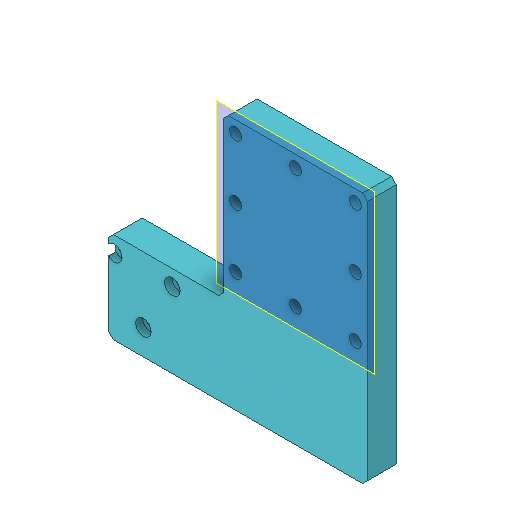
# Autodesk Inventor part: cellSTORM_Base_v0_R1
Saved by Autodesk Inventor 2022 (Build 260153000, 153)
## iProperties
Created: 2019-10-29
Part Number: cellSTORM_Base_v0_R1
Material: Generic
Document SubType Name: Modeling
Designer: diederichbenedict
Density: 1 g/cm^3
Appearance: Default
Sheet Metal Rule: Standard
Author: diederichbenedict
Autodesk Inventor part; units mm, degrees
ref_plane "YZ Plane" through (0, 0, 0) normal (1, 0, 0) x (0, 1, 0)
ref_plane "XZ Plane" through (0, 0, 0) normal (0, 1, 0) x (-1, 0, 0)
ref_plane "XY Plane" through (0, 0, 0) normal (0, 0, 1) x (1, 0, 0)
ref_plane "Arbeitsebene2" through (0, 0, 0) normal (0, 0, -1) x (0, 1, 0)
sketch "Skizze6" plane through (0, 0, 0) normal (0, 0, -1) x (0, 1, 0)
  circle A0 centre (0, 25) radius 1.95 projected
  circle A1 centre (-25, 0) radius 1.95 projected
  circle A2 centre (-25, -25) radius 1.95 projected
  circle A3 centre (25, 25) radius 1.95 projected
  circle A4 centre (25, -25) radius 1.95 projected
  circle A5 centre (-25, 25) radius 1.95 projected
  circle A6 centre (25, 0) radius 1.95 projected
  circle A7 centre (0, -25) radius 1.95 projected
  line L0 (-28, 30) -> (-30, 28) projected
  line L1 (-30, 28) -> (-30, -28) projected
  line L2 (-30, -28) -> (-28, -30) projected
  line L3 (-28, -30) -> (28, -30) projected
  line L4 (28, -30) -> (30, -28) projected
  line L5 (30, -28) -> (30, 28) projected
  line L6 (30, 28) -> (28, 30) projected
  line L7 (28, 30) -> (-28, 30) projected
  line L8 (-40.5166, -48.4344) -> (-70.5166, -48.4344) construction
  line L9 (-70.5166, -48.4344) -> (-70.5166, -78.4344) construction
  line L10 (-70.5166, -78.4344) -> (-40.5166, -78.4344) construction
  line L11 (-40.5166, -78.4344) -> (-40.5166, -48.4344) construction
  line L12 (-40.5166, -48.4344) -> (-70.5166, -78.4344) construction
  line L13 (-70.5166, -48.4344) -> (-40.5166, -78.4344) construction
  line L14 (-75, -48) -> (-45, -48)
  line L15 (-45, -48) -> (-45, -78)
  line L16 (-45, -78) -> (-75, -78)
  line L17 (-75, -78) -> (-75, -48)
  line L18 (-75, -48) -> (-45, -78) construction
  line L19 (-45, -48) -> (-75, -78) construction
  line L20 (-45, -48) -> (-30, -48)
  line L21 (-30, -48) -> (-30, -28)
  line L22 (-45, -78) -> (0, -78)
  line L23 (0, -78) -> (0, -30)
  circle A8 centre (-55.5095, -63.317) radius 8.4793 projected
  line L24 (-28, 30) -> (-75, 30)
  line L25 (-75, 30) -> (-75, -48)
  line L26 (-28, -30) -> (-45, -30)
  line L27 (-45, -30) -> (-45, -48)
  line L28 (-45, -78) -> (-37, -78)
  line L29 (-37, -78) -> (-37, -48)
  line L30 (-37, -48) -> (-45, -48)
  line L31 (-45, -48) -> (-45, -78)
  line L32 (-45, -30) -> (-37, -30)
  line L33 (-37, -30) -> (-37, -48)
  line L34 (-37, -48) -> (-45, -48)
  line L35 (-45, -48) -> (-45, -30)
  point P0 (0, 0)
  point P1 (-55.5166, -63.4344)
  point P2 (-60, -63)
  dimension "d10" = 30
  dimension "d11" = 30
  dimension "d12" = 30
  dimension "d13" = 30
  dimension "d14" = 45
  dimension "d15" = 18
  dimension "d28" = 8
  constraints: 56 end point, 9 parallel, 8 horizontal, 7 perpendicular, 5 midpoint, 1 point on line
  measures "d10" distance of L10.end L9.end
  measures "d11" distance of L9.end L8.end
  measures "d12" distance of L15.end L16.end
  measures "d13" distance of L14.end L15.end
  measures "d14" distance between parallel lines of L15 L23
  measures "d15" distance between parallel lines of L3 L20
  measures "d28" distance of L30.end L29.end
extrude "Extrusion1" add sketch "Skizze6" along normal blind 12 contours L7 L6 L5 L4 L3 L2 L1 L0 | L0 L1 L21 L26 L27 L14 L25 L24 | L2 L26 L21 | L14 L15 L16 L17 | L20 L29 L22 L15 | L27 L26 L33 L20 | A8
chamfer "Fase1" distance 2 angle 45 4 edges at (-78, -75, -6) (30, -75, -6) (-30, -37, -6) (-78, -37, -6)
sketch "Skizze7" plane through (0, 0, -12) normal (0, 0, -1) x (-1, 0, 0)
  line L0 (30, -35) -> (30, 28) projected
  line L1 (30, 28) -> (28, 30) projected
  line L2 (28, 30) -> (-28, 30) projected
  line L3 (-28, 30) -> (-30, 28) projected
  line L4 (-30, 28) -> (-30, -73) projected
  circle A0 centre (25, 0) radius 1.95 projected
  circle A1 centre (0, 25) radius 1.95 projected
  circle A2 centre (-25, -25) radius 1.95 projected
  circle A3 centre (25, 25) radius 1.95 projected
  circle A4 centre (-25, 25) radius 1.95 projected
  circle A5 centre (25, -25) radius 1.95 projected
  circle A6 centre (0, -25) radius 1.95 projected
  circle A7 centre (-25, 0) radius 1.95 projected
  line L5 (78, -73) -> (76, -75) projected
  line L6 (-28, -75) -> (76, -75) projected
  line L7 (-28, -75) -> (-30, -73) projected
  line L8 (78, -73) -> (78, -39) projected
  line L9 (76, -37) -> (32, -37) projected
  line L10 (76, -37) -> (78, -39) projected
  line L11 (30, -35) -> (32, -37) projected
  point P0 (0, 0)
hole "Bohrung2" at (-25, 25, -12) at (-25, 0, -12) at (-25, -25, -12) at (25, -25, -12) at (25, 0, -12) at (25, 25, -12) at (0, 25, -12) at (0, -25, -12) direction (0, 0, 1) diameter 5 end through all counterbore diameter 8 counterbore depth 5
sketch "Skizze8" plane through (0, 0, 0) normal (0, 0, 1) x (1, 0, 0)
  circle A0 centre (-63.4834, -64.233) radius 2.95 projected
  circle A1 centre (-75.6078, -43.5) radius 2.95 projected
  circle A2 centre (-51.3591, -43.5) radius 2.95 projected
  point P0 (0, 0)
hole "Bohrung3" at (-51.3591, -43.5, 0) at (-63.4834, -64.233, 0) at (-75.6078, -43.5, 0) direction (0, 0, -1) diameter 2.8 end through all counterbore diameter 6.5 counterbore depth 3
equation "\"BendRadius\" = Thickness"
equation "\"BendReliefWidth\" = Thickness"
equation "\"BendReliefDepth\" = 0.5 * Thickness"
equation "\"CornerReliefSize\" = 4 * Thickness"
equation "\"MinimumRemnant\" = 2 * Thickness"
equation "\"TransitionRadius\" = BendRadius"
equation "\"JacobiRadiusSize\" = Thickness"
equation "\"GapSize\" = Thickness"
equation "\"Thickness\" = 0.5"
